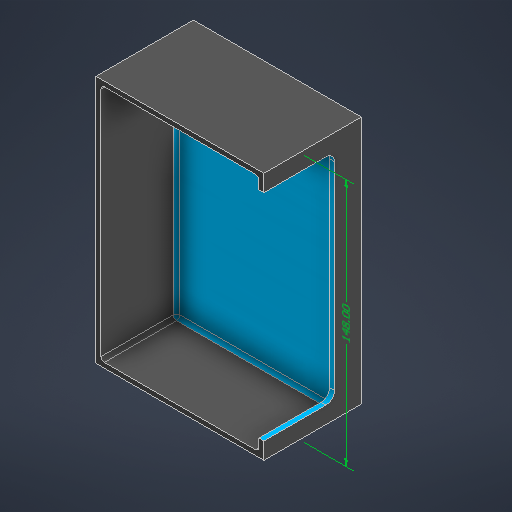
# Autodesk Inventor part: canecaCollision
Saved by Autodesk Inventor 2026.1 (Build 301233000, 233)
## iProperties
Created: 2025-04-25
Part Number: canecaCollision
Material: ABS NEGRO 4DLAB
Document SubType Name: Modeling
Designer: Joho_
Density: 0.894 g/cm^3
Appearance: Genérico
Mass: 120.072 g
Surface Area: 654.957 cm^2
Volume: 134.308 cm^3
Author: Joho_
## iProperties of the stored document _3DPrint.ipt
Created: 2025-04-28
Part Number: _3DPrint
Material: Genérico
Document SubType Name: Modeling
Designer: Joho_
Density: 1 g/cm^3
Appearance: Valor por defecto
Author: Joho_
Autodesk Inventor part; units mm, degrees
ref_plane "XZ Plane" through (0, 0, 0) normal (0, 1, 0) x (-1, 0, 0)
sketch "Boceto1" plane through (0, 0, 0) normal (0, 0, 1) x (1, 0, 0)
  circle A0 centre (80, 128) radius 1.85
  circle A1 centre (20, 128) radius 1.85
  circle A2 centre (80, 20) radius 1.85
  circle A3 centre (20, 20) radius 1.85
  line L0 (0, 0) -> (100, 0)
  line L1 (0, 148) -> (0, 0)
  line L2 (97, 3) -> (3, 3)
  line L3 (3, 3) -> (3, 145)
  line L4 (97, 145) -> (97, 3)
  line L5 (100, 0) -> (100, 148)
  line L6 (3, 145) -> (97, 145)
  line L7 (100, 148) -> (0, 148)
  circle A4 centre (20, 128) radius 4
  circle A5 centre (80, 128) radius 4
  circle A6 centre (20, 20) radius 4
  circle A7 centre (80, 20) radius 4
  dimension "d0" = 8
  dimension "d1" = 8
  dimension "d2" = 8
  dimension "d3" = 8
  dimension "d30" = 3.7
  dimension "d31" = 3.7
  dimension "d32" = 3.7
  dimension "d33" = 3.7
  constraints: 16 end point, 8 centre point, 4 coincident
  measures "d0" diameter of A4
  measures "d1" diameter of A5
  measures "d2" diameter of A6
  measures "d3" diameter of A7
  measures "d30" diameter of A1
  measures "d31" diameter of A3
  measures "d32" diameter of A0
  measures "d33" diameter of A2
extrude "base1" add sketch "Boceto1" against normal blind 10 contours A0 | A1 | A2 | A3 | L1 L7 L5 L0 | L2 L3 L6 L4 | A4 | A5 | A6 | A7
extrude "base2" add sketch "Boceto1" along normal blind 3 contours A0 | A1 | A2 | A3 | L2 L3 L6 L4 | A4 | A5 | A6 | A7
extrude "Extrusión3" add sketch "Boceto1" along normal blind 48 contours L1 L7 L5 L0
sketch "Boceto2" plane through (100, 0, -10) normal (1, 0, 0) x (0, 0, -1)
  line L0 (-16, 10) -> (-86, 10)
  line L1 (-86, 10) -> (-86, 138)
  line L2 (-86, 138) -> (-16, 138)
  line L3 (-16, 138) -> (-16, 10)
  point P0 (-3, 0)
  point P1 (-51, 74)
  dimension "d10" = 70
  dimension "d11" = 128
  constraints: 8 end point
  measures "d10" distance of L1.end L2.end
  measures "d11" distance of L0.end L1.end
extrude "Extrusión4" cut sketch "Boceto2" against normal blind 48
sketch "Boceto3" plane through (0, 0, 0) normal (1, 0, 0) x (0, 1, 0)
  point P0 (0, 0)
fillet "Empalme2" radius 2 8 edges at (3, 3, 25.5) (50, 3, 3) (3, 74, 3) (3, 145, 25.5) (50, 145, 3) (97, 145, 25.5) (97, 74, 3) (97, 3, 25.5)
fillet "Empalme2" radius 5 2 edges at (98.5, 138, 6) (98.5, 10, 6)
ref_plane "Plano de trabajo1" through (120, 0, 0) normal (1, 0, 0) x (0, 1, 0)
sketch "Boceto4" plane through (120, 0, 0) normal (1, 0, 0) x (0, 1, 0)
  arc A0 (0, 2.8284) -> (0.5858, 1.4142) centre (2, 2.8284) ccw
  line L0 (0, 48) -> (0, 2.8284)
  line L1 (5, -3) -> (0.5858, 1.4142)
  line L2 (5, -3) -> (143, -3)
  line L3 (143, -3) -> (147.4142, 1.4142)
  line L4 (148, 2.8284) -> (148, 48)
  arc A1 (147.4142, 1.4142) -> (148, 2.8284) centre (146, 2.8284) ccw
  line L5 (146, 48) -> (148, 48)
  line L6 (143, 48) -> (146, 48)
  line L7 (5, 48) -> (143, 48)
  line L8 (2, 48) -> (5, 48)
  line L9 (0, 48) -> (2, 48)
  arc A2 (10, 43) -> (5, 48) centre (5, 43) ccw
  line L10 (10, 18) -> (10, 43)
  arc A3 (10, 18) -> (15, 13) centre (15, 18) ccw
  line L11 (133, 13) -> (15, 13)
  arc A4 (133, 13) -> (138, 18) centre (133, 18) ccw
  line L12 (138, 43) -> (138, 18)
  arc A5 (143, 48) -> (138, 43) centre (143, 43) ccw
  point P0 (0, 0)
  constraints: 26 end point, 12 point on circle, 6 centre point
sketch "Boceto5" plane through (0, 0, 0) normal (0, 1, 0) x (-1, 0, 0)
  arc A0 (0, 46.5) -> (-1.5, 48) centre (-1.5, 46.5) ccw
  line L0 (-2, 48) -> (-1.5, 48)
  line L1 (-2, 48) -> (-98, 48)
  line L2 (0, 46.5) -> (0, 2.8284)
  arc A1 (-98.5, 48) -> (-100, 46.5) centre (-98.5, 46.5) ccw
  line L3 (-98.5, 48) -> (-98, 48)
  line L4 (-100, 2.8284) -> (-100, 46.5)
  arc A2 (-100, 2.8284) -> (-99.4142, 1.4142) centre (-98, 2.8284) ccw
  line L5 (-95, -3) -> (-99.4142, 1.4142)
  line L6 (-5, -3) -> (-95, -3)
  arc A3 (-0.5858, 1.4142) -> (0, 2.8284) centre (-2, 2.8284) ccw
  line L7 (-5, -3) -> (-0.5858, 1.4142)
  point P0 (0, 0)
  constraints: 16 end point, 8 point on circle, 4 centre point
extrude "Extrusión5" cut sketch "Boceto1" along normal blind 2 contours A0 | A1 | A2 | A3
ref_plane "Plano de trabajo2" through (0, 0, -3) normal (0, 0, 1) x (1, 0, 0)
sketch "Boceto6" plane through (0, 0, -3) normal (0, 0, 1) x (1, 0, 0)
  circle A0 centre (20, 128) radius 2
  circle A1 centre (20, 128) radius 2.3
  circle A2 centre (20, 20) radius 0.35 projected
  circle A3 centre (20, 20) radius 2.3
  circle A4 centre (80, 20) radius 0.35 projected
  circle A5 centre (80, 20) radius 2.3
  circle A6 centre (80, 128) radius 0.35 projected
  circle A7 centre (80, 128) radius 2.3
  point P0 (0, 0)
  dimension "d29" = 4.6
  dimension "d34" = 4.6
  dimension "d35" = 4.6
  dimension "d36" = 4.6
  constraints: 5 centre point, 4 coincident
  measures "d29" diameter of A1
  measures "d34" diameter of A3
  measures "d35" diameter of A5
  measures "d36" diameter of A7
extrude "Extrusión6" [suppressed]
